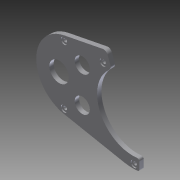
# Autodesk Inventor part: connected plate
Saved by Autodesk Inventor 2012 (Build 160160000, 160)
## iProperties
Created: 2012-01-30
Part Number: connected plate
Material: Default
Document SubType Name: Modeling
Designer: Antonella Wilby
Density: 1 g/cm^3
Author: Antonella Wilby
Autodesk Inventor part; units mm, degrees
ref_plane "YZ Plane" through (0, 0, 0) normal (1, 0, 0) x (0, 1, 0)
ref_plane "XZ Plane" through (0, 0, 0) normal (0, 1, 0) x (-1, 0, 0)
ref_plane "XY Plane" through (0, 0, 0) normal (0, 0, 1) x (1, 0, 0)
sketch "Sketch1" plane through (0, 0, 0) normal (0, 0, 1) x (1, 0, 0)
  circle A0 centre (0, 0) radius 50.8 construction
  arc A1 (-100.3903, 49.8474) -> (-100.3903, -49.8474) centre (-90.5988, 0) ccw
  line L0 (-100.3903, 49.8474) -> (-44.1544, 60.8938)
  line L1 (-100.3903, -49.8474) -> (-13.1573, -66.9825)
  circle A2 centre (-74.0404, 25.4) radius 11.1125
  circle A3 centre (-74.0404, -25.4) radius 11.1125
  line L2 (-179.8386, 0) -> (89.2398, 0) projected
  line L3 (0, -95.9117) -> (0, 94.8458) projected
  line L4 (9.525, -55.1985) -> (9.525, -64.777)
  arc A4 (-13.1573, -66.9825) -> (6.6598, -67.9369) centre (0, 0) ccw
  arc A5 (-34.7181, 39.2314) -> (5.9871, -52.0443) centre (0, 0) ccw
  arc A6 (9.525, -55.1985) -> (5.9871, -52.0443) centre (6.35, -55.1985) ccw
  arc A7 (6.6598, -67.9369) -> (9.525, -64.777) centre (6.35, -64.777) ccw
  circle A8 centre (-107.95, 0) radius 14.2875
  line L5 (-107.95, -14.2875) -> (-107.95, 14.2875) construction
  line L6 (0, 0) -> (-43.7877, 43.7877) construction
  line L7 (-32.9808, 46.2166) -> (-36.9849, 56.8928)
  arc A9 (-36.9849, 56.8928) -> (-44.1544, 60.8938) centre (-42.9305, 54.6628) ccw
  arc A10 (-34.7181, 39.2314) -> (-32.9808, 46.2166) centre (-38.9264, 43.9867) ccw
  point P0 (-38.8745, 61.9309)
  point P1 (9.525, 51.5143)
  point P2 (9.525, 67.5947)
  point P3 (9.525, -51.5143)
  point P4 (9.525, -67.5947)
  point P5 (0, 52.3875)
  point P6 (-31.3803, 41.9491)
  dimension "d0" = 101.6
  dimension "d9" = 22.225
  dimension "d13" = 1.5875
  dimension "d16" = 15.875
  dimension "d28" = 50.8
  dimension "d38" = 28.575
  dimension "d39" = 107.95
  dimension "d40" = 45
  dimension "d41" = 61.9252
  dimension "d51" = 6.35
  constraints: 20 point on circle, 12 end point, 11 centre point, 11 tangent, 7 point on line, 3 coincident, 1 equal radius, 1 horizontal alignment, 1 midpoint
  measures "d0" diameter of A0
  measures "d9" diameter of A2
  measures "d13" radial gap between concentric circles of A5 A0
  measures "d16" radial gap between concentric circles of A5 A4
  measures "d28" radius of A1
  measures "d38" diameter of A8
  measures "d39" distance between parallel lines of L5 L3
  measures "d40" angle of L3 L6
  measures "d41" distance of L6.start L6.end
  measures "d51" radius of A9
extrude "Extrusion1" add sketch "Sketch1" along normal mid plane 6.35 contours L0 A9 L7 A10 A5 L2 A8 A1 | L2 A8 A5 L3 A4 L1 A1 | L3 A5 A6 L4 A7 A4
sketch "Sketch2" plane through (0, 0, 3.175) normal (0, 0, 1) x (1, 0, 0)
  line L0 (-171.5836, 0) -> (39.7098, 0) projected
  line L1 (0, -94.2975) -> (0, 87.9475) projected
  point P0 (1.5875, 61.9125)
  point P1 (1.5875, -61.9125)
  dimension "d19" = 1.5875
  dimension "d20" = 61.9125
  constraints: 1 symmetric about line
  measures "d19" distance from line of point (1.587, 61.913) L1
  measures "d20" distance from line of point (1.587, 61.913) L0
hole "Hole1" at (1.5875, 61.9125, 3.175) at (1.5875, -61.9125, 3.175) direction (0, 0, -1) diameter 5.1054 end through all counterbore diameter 9.779 counterbore depth 1.5875 clearance for "Flat Head Machine Screw (82)" size "#10" standard "Ansi Unified Screw Threads"
sketch "Sketch3" plane through (0, 0, 3.175) normal (0, 0, 1) x (1, 0, 0)
  line L0 (9.525, 64.777) -> (9.525, 55.1985) projected
  line L1 (-100.3903, -49.8474) -> (-100.3903, 49.8474) construction
  line L2 (-171.5836, 0) -> (39.7098, 0) projected
  line L3 (0, -94.8704) -> (0, 91.3849) projected
  point P0 (-100.3903, 42.8625)
  point P1 (-100.3903, -42.8625)
  dimension "d29" = 42.8625
  constraints: 2 end point, 1 parallel, 1 point on line, 1 symmetric about line
  measures "d29" distance from line of point (-100.39, 42.862) L2
hole "Hole2" at (-100.3903, 42.8625, 3.175) at (-100.3903, -42.8625, 3.175) direction (0, 0, -1) diameter 5.1054 end through all counterbore diameter 9.779 counterbore depth 1.5875 clearance for "Flat Head Machine Screw (82)" size "#10" standard "Ansi Unified Screw Threads"
sketch "Sketch4" plane through (0, 0, 3.175) normal (0, 0, 1) x (1, 0, 0)
  arc A0 (-34.7181, 39.2314) -> (5.9871, -52.0443) centre (0, 0) ccw projected
  line L0 (0, 0) -> (-43.7877, 43.7877) construction
  line L1 (-171.5836, 0) -> (39.7098, 0) projected
  line L2 (0, -94.1176) -> (0, 86.8679) projected
  point P0 (5.9871, 52.0443)
  dimension "d42" = 61.9252
  dimension "d43" = 45
  constraints: 2 end point
  measures "d42" distance of L0.start L0.end
  measures "d43" angle of L2 L0
hole "Hole3" at (-43.7877, 43.7877, 3.175) direction (0, 0, -1) diameter 5.1054 end through all counterbore diameter 9.779 counterbore depth 1.5875 clearance for "Flat Head Machine Screw (82)" size "#10" standard "Ansi Unified Screw Threads"
body "Solid1"
